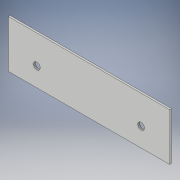
# Autodesk Inventor part: Panel_5x17cm
Saved by Autodesk Inventor 2019 (Build 230136000, 136)
## iProperties
Created: 2018-10-31
Part Number: Panel_5x17cm
Material: Generic
Document SubType Name: Modeling
Designer: nomol
Density: 1 g/cm^3
Appearance: Default
Author: nomol
Autodesk Inventor part; units mm, degrees
ref_plane "YZ Plane" through (0, 0, 0) normal (1, 0, 0) x (0, 1, 0)
ref_plane "XZ Plane" through (0, 0, 0) normal (0, 1, 0) x (-1, 0, 0)
ref_plane "XY Plane" through (0, 0, 0) normal (0, 0, 1) x (1, 0, 0)
sketch "Sketch1" plane through (0, 0, 0) normal (0, 0, 1) x (1, 0, 0)
  line L0 (0, 0) -> (170, 0)
  line L1 (170, 0) -> (170, 50)
  line L2 (170, 50) -> (0, 50)
  line L3 (0, 50) -> (0, 0)
  dimension "d0" = 170
  dimension "d1" = 50
  constraints: 8 end point, 2 parallel, 1 horizontal, 1 perpendicular
  measures "d0" distance of L1.end L2.end
  measures "d1" distance of L0.end L1.end
extrude "Extrusion1" add sketch "Sketch1" along normal blind 2
sketch "Sketch2" plane through (0, 0, 2) normal (0, 0, 1) x (1, 0, 0)
  circle A0 centre (30, 20) radius 3.57
  circle A1 centre (140, 20) radius 3.57
  line L0 (0, 0) -> (170, 0) projected
  line L1 (0, 50) -> (0, 0) projected
  line L2 (170, 0) -> (170, 50) projected
  dimension "d4" = 7.14
  dimension "d5" = 7.14
  dimension "d6" = 20
  dimension "d7" = 30
  dimension "d8" = 30
  dimension "d9" = 20
  constraints: 2 centre point
  measures "d4" diameter of A0
  measures "d5" diameter of A1
  measures "d6" distance from line of L0 A0.centre
  measures "d7" distance from line of L1 A0.centre
  measures "d8" distance from line of L2 A1.centre
  measures "d9" distance from line of L0 A1.centre
extrude "Extrusion2" cut sketch "Sketch2" against normal up to next
body "Solid1"
